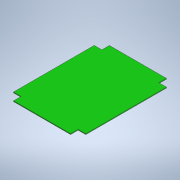
# Autodesk Inventor part: Mock Module PCB
Saved by Autodesk Inventor 2022 (Build 260153000, 153)
## iProperties
Created: 2021-07-19
Part Number: Mock Module PCB
Material: Generic
Document SubType Name: Modeling
Designer: Caleb
Density: 1 g/cm^3
Appearance: Default
Author: Caleb
Autodesk Inventor part; units mm, degrees
ref_plane "YZ Plane" through (0, 0, 0) normal (1, 0, 0) x (0, 1, 0)
ref_plane "XZ Plane" through (0, 0, 0) normal (0, 1, 0) x (-1, 0, 0)
ref_plane "XY Plane" through (0, 0, 0) normal (0, 0, 1) x (1, 0, 0)
sketch "Sketch1" plane through (0, 0, 0) normal (0, 1, 0) x (-1, 0, 0)
  line L0 (-21.3, 28.25) -> (21.3, 28.25)
  line L1 (21.3, 28.25) -> (21.3, -28.25)
  line L2 (21.3, -28.25) -> (-21.3, -28.25)
  line L3 (-21.3, -28.25) -> (-21.3, 28.25)
  line L4 (-21.3, 28.25) -> (21.3, -28.25) construction
  line L5 (21.3, 28.25) -> (-21.3, -28.25) construction
  point P0 (0, 0)
  dimension "d0" = 42.6
  dimension "d1" = 56.5
  constraints: 12 end point, 2 midpoint, 2 parallel, 1 horizontal, 1 perpendicular
  measures "d0" distance of L0.start L0.end
  measures "d1" distance of L0.end L1.end
extrude "Extrusion1" add sketch "Sketch1" along normal blind 0.5
sketch "Sketch5" plane through (0, 0.5, 0) normal (0, 1, 0) x (1, 0, 0)
  line L0 (21.3, 28.25) -> (-21.3, 28.25) projected
  line L1 (-21.3, 28.25) -> (-16.8, 28.25)
  line L2 (-16.8, 28.25) -> (-16.8, 23.8)
  line L3 (-16.8, 23.8) -> (-21.3, 23.8)
  line L4 (-21.3, 23.8) -> (-21.3, 28.25)
  line L5 (21.3, 28.25) -> (16.8, 28.25)
  line L6 (16.8, 28.25) -> (16.8, 23.8)
  line L7 (16.8, 23.8) -> (21.3, 23.8)
  line L8 (21.3, 23.8) -> (21.3, 28.25)
  line L9 (-21.3, -28.25) -> (21.3, -28.25) projected
  line L10 (21.3, -28.25) -> (16.8, -28.25)
  line L11 (16.8, -28.25) -> (16.8, -23.8)
  line L12 (16.8, -23.8) -> (21.3, -23.8)
  line L13 (21.3, -23.8) -> (21.3, -28.25)
  line L14 (-21.3, -28.25) -> (-16.8, -28.25)
  line L15 (-16.8, -28.25) -> (-16.8, -23.8)
  line L16 (-16.8, -23.8) -> (-21.3, -23.8)
  line L17 (-21.3, -23.8) -> (-21.3, -28.25)
  point P0 (0, 0)
  dimension "d23" = 4.5
  dimension "d24" = 4.45
  dimension "d25" = 4.45
  dimension "d26" = 4.45
  dimension "d27" = 4.45
  dimension "d28" = 4.5
  dimension "d29" = 4.5
  dimension "d30" = 4.5
  constraints: 32 end point, 8 parallel, 4 horizontal, 4 perpendicular
  measures "d23" distance of L2.end L3.end
  measures "d24" distance of L1.end L2.end
  measures "d25" distance of L14.end L15.end
  measures "d26" distance of L10.end L11.end
  measures "d27" distance of L5.end L6.end
  measures "d28" distance of L6.end L7.end
  measures "d29" distance between parallel lines of L11 L13
  measures "d30" distance of L15.end L16.end
extrude "Extrusion2" cut sketch "Sketch5" against normal through all
equation "\"d25\" = d24"
equation "\"d26\" = d24"
equation "\"d27\" = d24"
equation "\"d28\" = d23"
equation "\"d29\" = d23"
equation "\"d30\" = d23"
body "Solid1"
